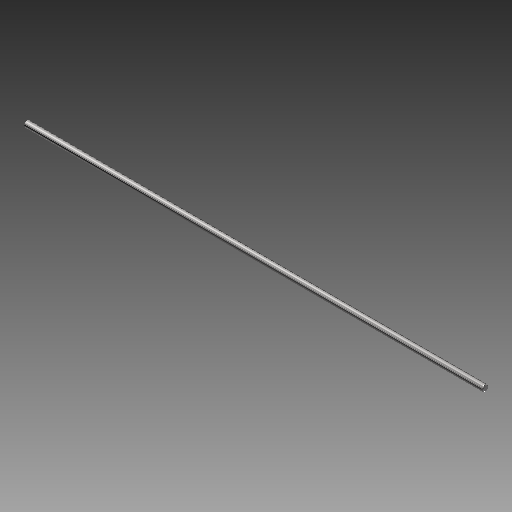
# Autodesk Inventor part: Shaft
Saved by Autodesk Inventor 2018 (Build 220112000, 112)
## iProperties
Created: 2018-08-06
Part Number: Shaft
Material: Steel, Mild
Document SubType Name: Modeling
Designer: Cole Tucker
Density: 7.85 g/cm^3
Appearance: Semi-Polished
Mass: 908.021 g
Surface Area: 366.222 cm^2
Volume: 115.671 cm^3
CustomPartVersion: 1
Author: Cole Tucker
Autodesk Inventor part; units mm, degrees
ref_plane "Start Plane" through (0, 0, 0) normal (1, 0, 0) x (0, 1, 0)
ref_plane "XZ Plane" through (0, 0, 0) normal (0, 1, 0) x (-1, 0, 0)
ref_plane "XY Plane" through (0, 0, 0) normal (0, 0, 1) x (1, 0, 0)
sketch "Main Sketch" plane through (0, 0, 0) normal (0, 0, 1) x (1, 0, 0)
  line L0 (0, 0) -> (914.4, 0)
  line L1 (0, 0) -> (0, 6.35)
  line L2 (914.4, 6.35) -> (914.4, 0)
  line L3 (0, 6.35) -> (914.4, 6.35)
  dimension "d3" = 12.7
  constraints: 8 end point, 3 horizontal, 2 vertical
  measures "d3" diameter of L3 L0
revolve "Revolution1" add sketch "Main Sketch" angle 360 about axis through (0, 0, 0) along (1, 0, 0)
chamfer "Chamfer1" distance 2.54 angle 45 1 edges at (0, -6.35, 0) measured on face at (609.6, 6.3294, -0.511)
fillet "Fillet1" radius 2.54 1 edges at (914.4, -6.35, 0)
body "Solid1"
